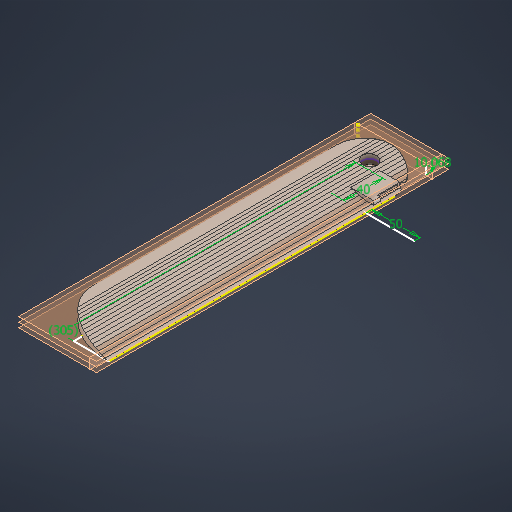
# Autodesk Inventor part: wing ready for torsiom WITH COOKIE
Saved by Autodesk Inventor 2026.2 (Build 302298010, 298A)
## iProperties
Created: 2026-05-08
Part Number: wing ready for torsiom WITH COOKIE
Material: Generic
Document SubType Name: Modeling
Designer: Jake
Density: 1 g/cm^3
Appearance: Default
Autodesk Inventor part; units mm, degrees
sketch "CLARK_Y_73mm" plane through (0, 0, 0) normal (0, 0, 1) x (1, 0, 0)
  line L0 (18.25, 9.709) -> (21.9, 9.928)
  line L1 (21.9, 9.928) -> (25.55, 9.9645)
  line L2 (25.55, 9.9645) -> (29.2, 9.855)
  line L3 (29.2, 9.855) -> (32.85, 9.6068)
  line L4 (32.85, 9.6068) -> (36.5, 9.2272)
  line L5 (36.5, 9.2272) -> (40.15, 8.7308)
  line L6 (40.15, 8.7308) -> (43.8, 8.1176)
  line L7 (43.8, 8.1176) -> (47.45, 7.4095)
  line L8 (47.45, 7.4095) -> (51.1, 6.5919)
  line L9 (51.1, 6.5919) -> (54.75, 5.6794)
  line L10 (54.75, 5.6794) -> (58.4, 4.6647)
  line L11 (58.4, 4.6647) -> (62.05, 3.5697)
  line L12 (62.05, 3.5697) -> (65.7, 2.3944)
  line L13 (65.7, 2.3944) -> (69.35, 1.168)
  line L14 (69.35, 1.168) -> (73, 0)
  line L15 (73, 0) -> (69.35, 0)
  line L16 (69.35, 0) -> (65.7, 0)
  line L17 (65.7, 0) -> (62.05, 0)
  line L18 (62.05, 0) -> (58.4, 0)
  line L19 (58.4, 0) -> (51.1, 0)
  line L20 (51.1, 0) -> (43.8, 0)
  line L21 (43.8, 0) -> (36.5, 0)
  line L22 (36.5, 0) -> (29.2, 0)
  line L23 (29.2, 0) -> (21.9, 0)
  line L24 (21.9, 0) -> (14.6, 0)
  line L25 (14.6, 0) -> (7.3, 0)
  line L26 (7.3, 0) -> (3.65, 0)
  line L27 (3.65, 0) -> (2.19, 0)
  line L28 (0.365, 0.511) -> (0.1825, 0.9271)
  arc A0 (0.1399, 1.8528) -> (0.365, 0.511) centre (1.7657, 1.4357) ccw
  line L29 (0.365, 0.511) -> (0.5265, 0.2899) construction
  line L30 (0.5265, 0.2899) -> (0.9522, 0) construction
  line L31 (0.9522, 0) -> (2.19, 0) construction
  spline S0 degree 3 poles (0.365, 0.511) (0.5265, 0.2899) (0.9522, 0) (2.19, 0) knots 1 1 1 1 2 2 2 2
  spline S1 degree 4 poles (0.1399, 1.8528) (0.2619, 2.7657) (0.8334, 3.4682) (1.0375, 4.4233) (3.8017, 6.4908) (5.5937, 7.0607) (8.27, 8.1821) (13.8932, 9.2359) (15.4936, 9.4158) (18.25, 9.709) knots 0 0 0 0 0 0.154503 0.263225 0.373674 0.500009 0.631398 1 1 1 1 1
  line L32 (-0.2816, -1.3009) -> (0.5615, 5.0066) construction
  arc A1 (1.0397, 3.9099) -> (0.4679, -0.3683) centre (4.1739, 1.3137) ccw construction
  point P0 (0.7298, 3.4456)
  point P1 (1.4608, 4.5019)
  point P2 (3.6506, 6.2246)
  point P3 (5.4755, 7.0495)
  point P4 (7.3004, 7.6919)
  point P5 (10.9503, 8.6122)
  point P6 (14.6001, 9.27)
  point P7 (2.1831, 0)
  constraints: 60 end point, 3 point on circle, 2 centre point, 2 midpoint, 1 horizontal, 14 other
extrude "Extrusion1" add sketch "CLARK_Y_73mm" along normal blind 330
ref_plane "Work Plane1" through (0, 10, 0) normal (0, 1, 0) x (-1, 0, 0)
sketch "Sketch3" plane through (0, 10, 0) normal (0, 1, 0) x (-1, 0, 0)
  line L0 (-0.365, 0) -> (-0.365, 330) projected
  line L1 (-0.365, 0) -> (-36.865, 0)
  line L2 (-2.1831, 0) -> (-73, 0) projected
  line L3 (-36.865, 0) -> (-36.865, 25)
  circle A0 centre (-36.865, 25) radius 7.5
  point P0 (0, 0)
  dimension "d3" = 36.5
  dimension "d4" = 25
  dimension "d5" = 90
  dimension "d6" = 15
  constraints: 4 end point, 1 centre point, 1 coincident, 1 perpendicular, 1 point on line
  measures "d3" distance of L0.start L1.end
  measures "d4" distance of L1.end L3.end
  measures "d5" angle of L1 L3
  measures "d6" diameter of A0
extrude "Extrusion2" cut sketch "Sketch3" against normal blind 10
sketch "Sketch4" plane through (0, 10, 0) normal (0, 1, 0) x (-1, 0, 0)
  line L0 (-0.0873, 0) -> (-0.365, 0) projected
  line L1 (-0.0873, 0) -> (-0.0873, 40)
  line L2 (-0.365, 0) -> (-0.365, 330) projected
  line L3 (-0.0873, 0) -> (39.9127, 0) construction
  line L4 (-2.1831, 0) -> (-73, 0) projected
  circle A0 centre (-36.865, 25) radius 7.5 projected
  line L5 (-36.865, 25) -> (-36.865, 0)
  arc A1 (-36.865, 0) -> (-0.0873, 40) centre (-38.0337, 37.982) ccw
  line L6 (-73, 0) -> (-73, 330) projected
  arc A2 (-73, 40) -> (-36.865, 0) centre (-35.055, 37.9569) ccw
  spline S0 degree 4 poles (-36.865, 0) (-53.2953, -17.7572) (-31.1868, -57.9375) (60.195, -74.7292) (77.3255, -11.4018) (105.6868, 69.3906) (-50.1321, 70.3306) (65.3998, 12.8936) (-0.0873, 40) knots 0 0 0 0 0 0.314626 0.457461 0.601529 0.730669 1 1 1 1 1
  spline S1 degree 4 poles (-73, 35.9137) (-95.9746, 88.4529) (-260.1854, -104.9165) (-4.2152, -29.3195) (-22.4351, -44.3111) knots 0 0 0 0 0 1 1 1 1 1
  point P0 (0, 0)
  point P1 (-0.1399, 0)
  point P2 (-39.6267, -26.5056)
  point P3 (0.9647, -54.7274)
  point P4 (53.8055, -50.0438)
  point P5 (78.9049, -7.651)
  point P6 (70.018, 46.6309)
  point P7 (17.5375, 53.9566)
  point P8 (23.1818, 36.5431)
  point P9 (-116.9525, 26.9734)
  point P10 (-128.3571, -25.384)
  point P11 (-43.6003, -43.3983)
  point P12 (-0.365, 32.9748)
  point P13 (-0.0873, 35.9641)
  dimension "d9" = 40
  dimension "d10" = 90
  dimension "d12" = 38
  dimension "d13" = 38
  constraints: 6 end point, 5 point on circle, 3 point on line, 2 centre point, 2 perpendicular, 1 horizontal, 1 parallel, 15 other
  measures "d9" distance of L0.start L1.end
  measures "d10" angle of L3 L1
  measures "d12" radius of A1
  measures "d13" radius of A2
extrude "Extrusion3" cut sketch "Sketch4" against normal blind 10 contours L1 A1 S0 S1 L2 L0 | S0 S1 L6 L4 | L4 L6 A2
sketch "Sketch5" plane through (0, 10, 0) normal (0, 1, 0) x (-1, 0, 0)
  line L0 (-0.365, 32.9748) -> (-0.365, 330) projected
  line L1 (-0.0873, 0) -> (-0.0873, 330) projected
  arc A0 (-0.365, 32.9748) -> (-0.0873, 36.6911) centre (-75.3602, 40.4479) ccw
  line L2 (-0.0873, 36.6911) -> (6.4562, 35.8991)
  line L3 (6.4562, 35.8991) -> (11.0519, -10.6221)
  line L4 (11.0519, -10.6221) -> (-6.6707, 1.2707)
  line L5 (-6.6707, 1.2707) -> (-0.6639, 29.6101)
  line L6 (-0.6639, 29.6101) -> (-0.365, 32.9748)
  point P0 (0, 0)
  constraints: 10 end point, 2 point on circle, 1 centre point, 1 point on line
extrude "Extrusion4" cut sketch "Sketch5" against normal blind 10
sketch "Sketch6" plane through (0, 10, 0) normal (0, 1, 0) x (-1, 0, 0)
  line L0 (-0.365, 32.9748) -> (-0.365, 330) projected
  line L1 (-73, 35.9137) -> (-73, 330) projected
  line L2 (-72.9868, 330) -> (-0.365, 330)
  line L3 (-0.365, 330) -> (0.0001, 330)
  arc A0 (0.0001, 260.001) -> (-72.9868, 330) centre (-69.9998, 260.0638) ccw
  line L4 (0.0001, 260.001) -> (37.973, 323.2416)
  line L5 (37.973, 323.2416) -> (8.7647, 382.8683)
  line L6 (8.7647, 382.8683) -> (-76.7506, 375.8481)
  line L7 (-76.7506, 375.8481) -> (-72.9868, 330)
  point P0 (0, 0)
  point P1 (-0.365, 260.001)
  dimension "d18" = 70
  dimension "d22" = 70
  constraints: 12 end point, 2 point on circle, 1 centre point, 1 collinear, 1 horizontal, 1 perpendicular, 1 point on line
  measures "d18" distance of L3.end point (-0.365, 260.001)
  measures "d22" radius of A0
extrude "Extrusion5" cut sketch "Sketch6" against normal blind 10 contours A0 L2 L0 | L0 L2 A0 L7 L6 L5 L4
ref_plane "Work Plane2" through (0, 0, 0) normal (0, 0, 1) x (1, 0, 0)
sketch "Sketch7" plane through (0, 0, 0) normal (0, 0, 1) x (1, 0, 0)
  line L0 (29.2, 9.855) -> (25.55, 9.9645) projected
  line L1 (25.55, 9.9645) -> (25.55, 5.0645)
  line L2 (2.1831, 0) -> (67.0128, 0) projected
  line L3 (25.55, 9.9645) -> (30.45, 9.9645) construction
  circle A0 centre (25.55, 5.0645) radius 3.5
  line L4 (58.4, 4.6647) -> (54.75, 5.6794) projected
  line L5 (54.75, 5.6794) -> (54.75, 0)
  line L6 (51.1, 6.5919) -> (47.45, 7.4095) projected
  line L7 (49.275, 7.0007) -> (49.275, 3.5007)
  line L8 (36.865, 0) -> (73, 0) projected
  line L9 (49.275, 7.0007) -> (52.775, 7.0007) construction
  circle A1 centre (49.275, 3.5007) radius 2.5
  point P0 (0, 0)
  dimension "d24" = 4.9
  dimension "d25" = 90
  dimension "d26" = 7
  dimension "d28" = 3.5
  dimension "d29" = 90
  dimension "d30" = 5
  constraints: 10 end point, 5 perpendicular, 2 centre point, 2 coincident, 2 horizontal, 1 midpoint, 1 point on line
  measures "d24" distance of L0.end L1.end
  measures "d25" angle of L1 L3
  measures "d26" diameter of A0
  measures "d28" distance of L7.start L7.end
  measures "d29" angle of L7 L9
  measures "d30" diameter of A1
extrude "Extrusion6" cut sketch "Sketch7" along normal blind 320 contours A1
extrude "Extrusion7" cut sketch "Sketch7" along normal blind 300 contours A0
ref_plane "Work Plane3" through (0, 0, 0) normal (0, 1, 0) x (-1, 0, 0)
sketch "Sketch8" plane through (0, 0, 0) normal (0, 1, 0) x (-1, 0, 0)
  arc A0 (-32.85, 31.3348) -> (-36.5, 32.4911) centre (-36.865, 25) ccw projected
  line L0 (-36.865, 25) -> (-36.5, 64.9983)
  line L1 (-36.5, 32.4911) -> (-36.5, 321.5273) projected
  line L2 (-36.5, 64.9983) -> (-73, 64.9983)
  line L3 (-73, 35.9137) -> (-73, 330) projected
  line L4 (-73, 64.9983) -> (-123, 64.9983)
  line L5 (-36.865, 25) -> (-36.865, 330)
  line L6 (-36.865, 330) -> (-73, 330)
  point P0 (0, 0)
  dimension "d36" = 40
  dimension "d37" = 50
  dimension "d38" = 305
  constraints: 10 end point, 2 horizontal, 2 point on line, 1 perpendicular, 1 vertical
  measures "d36" distance of L0.start L0.end
  measures "d37" distance of L2.end L4.end
  measures "d38" distance of L0.start L5.end
ref_plane "Work Plane4" through (70, 0, 0) normal (1, 0, 0) x (0, 1, 0)
sketch "Sketch11" plane through (70, 0, 0) normal (1, 0, 0) x (0, 1, 0)
  line L0 (1.0007, 27) -> (6.0007, 27) projected
  line L1 (6.0007, 27) -> (46.0007, 27) construction
  line L2 (4.0007, -21.5644) -> (8.0007, 27)
  line L3 (8.0007, 27) -> (4.0007, 27)
  line L4 (0, 25.3828) -> (0, 277.4101) projected
  line L5 (0, 27) -> (10, 27)
  line L6 (0, 27) -> (5, 27)
  line L7 (5, 27) -> (5, 57)
  line L8 (4.6647, 7.9734) -> (4.6647, 329.096) projected
  line L9 (5, 27) -> (35, 27) construction
  line L10 (5, 27) -> (7, 27)
  line L11 (6.0007, 2.7178) -> (6.0007, 320) projected
  line L12 (5, 27) -> (7, 27) construction
  line L13 (7, 27) -> (3, 27)
  line L14 (3, 27) -> (3, 57)
  line L15 (3, 57) -> (7, 57)
  line L16 (7, 57) -> (7, 27)
  point P0 (0, 0)
  point P1 (4.6647, 27)
  dimension "d49" = 10
  dimension "d50" = 5
  dimension "d51" = 30
  dimension "d52" = 90
  dimension "d53" = 2
  dimension "d54" = 0
  dimension "d55" = 4
  dimension "d56" = 30
  constraints: 26 end point, 5 horizontal, 3 parallel, 3 point on line, 2 equal length, 2 midpoint, 2 perpendicular, 1 other
  measures "d49" distance of L5.start L5.end
  measures "d50" distance of L5.start L6.end
  measures "d51" distance of L6.end L7.end
  measures "d52" angle of L9 L7
  measures "d53" distance of L6.end L10.end
  measures "d54" distance between parallel lines of L10 L12
  measures "d55" distance of L14.end L15.end
  measures "d56" distance of L13.end L14.end
extrude "Extrusion9" add sketch "Sketch11" against normal blind 24 contours L14 L15 L8 L0 | L8 L15 L7 L0 | L7 L15 L11 L0 | L11 L15 L16 L3
sketch "Sketch12" plane through (70, 0, 0) normal (1, 0, 0) x (0, 0, -1)
  line L0 (-27, 7) -> (-57, 7) projected
  line L1 (-27, 7) -> (-27, 5)
  line L2 (-27, 5.9855) -> (-27, 3) projected
  line L3 (-27, 5) -> (-29, 5)
  line L4 (-29, 5) -> (-55, 5)
  line L5 (-57, 3) -> (-57, 5.9855) projected
  line L6 (-55, 4) -> (-55, 6)
  line L7 (-55, 6) -> (-29, 6)
  line L8 (-29, 6) -> (-29, 4)
  line L9 (-29, 4) -> (-55, 4)
  line L10 (-55, 4) -> (-55, 6)
  point P0 (0, 0)
  dimension "d59" = 2
  dimension "d60" = 2
  dimension "d61" = 26
  dimension "d62" = 2
  dimension "d63" = 26
  dimension "d64" = 2
  constraints: 16 end point, 3 perpendicular, 2 parallel, 1 horizontal, 1 midpoint, 1 point on line, 1 vertical
  measures "d59" distance of L0.start L1.end
  measures "d60" distance of L1.end L3.end
  measures "d61" distance of L3.end L4.end
  measures "d62" distance of L6.start L6.end
  measures "d63" distance of L8.end L9.end
  measures "d64" distance of L7.end L8.end
extrude "Extrusion10" cut sketch "Sketch12" against normal blind 3
sketch "Sketch15" plane through (0, 10, 0) normal (0, 1, 0) x (-1, 0, 0)
  point P0 (0, 0)
sketch "Sketch16" plane through (70, 0, 0) normal (1, 0, 0) x (0, 0, -1)
  line L0 (-57, 6.5919) -> (-57, 7) projected
  line L1 (-57, 7) -> (-50, 7)
  line L2 (-50, 7) -> (-50, 3)
  line L3 (-50, 3) -> (-57, 3)
  line L4 (-57, 3) -> (-57, 7)
  point P0 (0, 0)
  dimension "d73" = 7
  dimension "d74" = 4
  constraints: 8 end point, 2 parallel, 1 horizontal, 1 perpendicular
  measures "d73" distance of L2.end L3.end
  measures "d74" distance of L1.end L2.end
extrude "Extrusion13" add sketch "Sketch16" along normal blind 3
sketch "Sketch17" plane through (70, 0, 0) normal (1, 0, 0) x (0, 0, -1)
  line L0 (-55, 6) -> (-50, 6) projected
  line L1 (-29, 4) -> (-50, 4) projected
  line L2 (-55, 6) -> (-49.1308, 6)
  line L3 (-49.1308, 6) -> (-49.1308, 4)
  line L4 (-49.1308, 4) -> (-55, 4)
  line L5 (-55, 4) -> (-55, 6)
  point P0 (0, 0)
  constraints: 8 end point, 2 parallel, 1 horizontal, 1 perpendicular, 1 point on line
extrude "Extrusion14" cut sketch "Sketch17" along normal blind 2
sketch "Sketch18" plane through (0, 10, 0) normal (0, 1, 0) x (-1, 0, 0)
  line L0 (-70, 27) -> (-70, 50) projected
  line L1 (-70, 27) -> (-70, 17.3992)
  line L2 (-71.4738, 50) -> (-71.4738, 21.5292)
  circle A0 centre (-71.4738, 21.5292) radius 5
  point P0 (0, 0)
  dimension "d79" = 10
  constraints: 4 end point, 2 vertical, 1 centre point, 1 coincident
  measures "d79" diameter of A0
extrude "Extrusion15" cut sketch "Sketch18" against normal blind 20
sketch "Sketch19" plane through (70, 0, 0) normal (1, 0, 0) x (0, 1, 0)
  line L0 (0, 0) -> (10.0684, 0)
  dimension "d82" = 10.0684
  constraints: 2 end point, 1 horizontal
  measures "d82" distance of L0.start L0.end
sketch "Sketch20" plane through (73, 0, 35.9137) normal (0, -1, 0) x (1, 0, 0)
  point P0 (-73, -35.9137)
sketch "Sketch21" plane through (0, 10, 0) normal (0, 1, 0) x (-1, 0, 0)
  point P0 (0, 0)
ref_plane "Work Plane5" through (0, 5, 0) normal (0, 1, 0) x (-1, 0, 0)
sketch "Sketch22" plane through (0, 5, 0) normal (0, 1, 0) x (-1, 0, 0)
  arc A0 (-32.85, 18.6652) -> (-32.85, 31.3348) centre (-36.865, 25) ccw projected
  circle A1 centre (-36.865, 25) radius 7.5
  point P0 (0, 0)
  constraints: 1 centre point, 1 coincident
body "Solid1"
